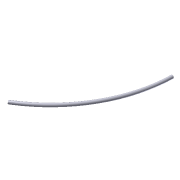
# Autodesk Inventor part: 2f2arc
Saved by Autodesk Inventor 2016 (Build 200138000, 138)
## iProperties
Company: HERA Project
Created: 2013-07-11
Part Number: 2f2arc
Material: Generic
Document SubType Name: Modeling
Designer: Dave
Density: 1 g/cm^3
Description: feed backplane pvc arc
Mass: 134.142 g
Surface Area: 939.016 cm^2
Volume: 134.142 cm^3
Appearance: Default
Author: David DeBoer
Autodesk Inventor part; units mm, degrees
ref_plane "YZ Plane" through (0, 0, 0) normal (1, 0, 0) x (0, 1, 0)
ref_plane "XZ Plane" through (0, 0, 0) normal (0, 1, 0) x (-1, 0, 0)
ref_plane "XY Plane" through (0, 0, 0) normal (0, 0, 1) x (1, 0, 0)
sketch "Sketch1" plane through (0, 0, 0) normal (0, 0, 1) x (1, 0, 0)
  circle A0 centre (596.9, -0.0117) radius 11
  line L0 (-252.1, 80.9625) -> (-252.1, -95.25)
  circle A1 centre (596.9, -0.0117) radius 9.38
  dimension "d6" = 22
  dimension "d7" = 849
  dimension "d9" = 1.62
  constraints: 2 centre point, 2 end point, 1 coincident, 1 vertical
  measures "d6" diameter of A0
  measures "d7" distance from line of L0 A0.centre
  measures "d9" radial gap between concentric circles of A1 A0
revolve "Revolution1" add sketch "Sketch1" angle 60 about axis through (-252.1, 80.9625, 0) along (0, -1, 0)
sketch "Sketch4" plane through (0, 0, 0) normal (0, 1, 0) x (-1, 0, 0)
  line L0 (-607.9, 0) -> (-585.9, 0) projected
  line L1 (-607.9, 0) -> (252.1, 0) construction
  line L2 (252.1, 0) -> (-596.7492, 16.0023) construction
  line L3 (-177.9, 744.7818) -> (-166.9, 725.7293) projected
  line L4 (252.1, 0) -> (-177.9, 744.7818) construction
  line L5 (252.1, 0) -> (-191.8616, 736.5447) construction
  arc A0 (-177.9, 744.7818) -> (-607.9, 0) centre (252.1, 0) ccw projected
  arc A1 (-596.7492, 16.0023) -> (-596.9, 0) centre (252.1, 0) ccw
  arc A2 (-172.4, 735.2556) -> (-186.183, 727.1238) centre (252.1, 0) ccw
  point P0 (0, 0)
  dimension "d10" = 860
  dimension "d12" = 1.08
  dimension "d13" = 1.08
  constraints: 8 end point, 5 point on circle, 3 point on line, 2 centre point, 1 coincident, 1 collinear
  measures "d10" distance of L0.start L1.end
  measures "d12" angle of L1 L2
  measures "d13" angle of L4 L5
sketch "Sketch5" plane through (596.9, -0.0117, 0) normal (0, 0, -1) x (-1, 0, 0)
  circle A0 centre (0, 0) radius 9.38
  circle A1 centre (0, 0) radius 11
  point P0 (596.9, 0.0117)
  constraints: 2 centre point, 1 coincident
sweep "Sweep1" cut profiles "Sketch5" path "Sketch4" path curves A1
sketch "Sketch6" plane through (172.4, -0.0117, 735.2556) normal (-0.8660254, 0, 0.5) x (0.5, 0, 0.8660254)
  circle A0 centre (0, 0) radius 9.38
  circle A1 centre (0, 0) radius 11
  point P0 (-722.95, 0.0117)
  constraints: 2 centre point, 1 coincident
sweep "Sweep2" cut profiles "Sketch6" path "Sketch4" path curves A2
body "Solid1"
